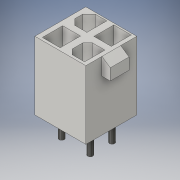
# Autodesk Inventor part: Molex_MiniFitJR_4Pos
Saved by Autodesk Inventor 2016 (Build 200138000, 138)
## iProperties
Created: 2016-09-29
Part Number: Molex_MiniFitJR_4Pos
Material: Generic
Document SubType Name: Modeling
Designer: jfixelle
Density: 1 g/cm^3
Appearance: White
Author: jfixelle
Autodesk Inventor part; units mm, degrees
ref_plane "YZ Plane" through (0, 0, 0) normal (1, 0, 0) x (0, 1, 0)
ref_plane "XZ Plane" through (0, 0, 0) normal (0, 1, 0) x (-1, 0, 0)
ref_plane "XY Plane" through (0, 0, 0) normal (0, 0, 1) x (1, 0, 0)
sketch "Sketch1" plane through (0, 0, 0) normal (0, 1, 0) x (-1, 0, 0)
  line L0 (4.9, 4.9) -> (-4.9, 4.9)
  line L1 (-4.9, 4.9) -> (-4.9, -4.9)
  line L2 (-4.9, -4.9) -> (4.9, -4.9)
  line L3 (4.9, -4.9) -> (4.9, 4.9)
  point P0 (0, 0)
  dimension "d0" = 9.8
  dimension "d1" = 9.8
  dimension "d2" = 4.9
  dimension "d3" = 4.9
  constraints: 8 end point, 2 parallel, 1 horizontal, 1 perpendicular
  measures "d0" distance of L2.end L0.start
  measures "d1" distance of L1.end L2.end
  measures "d2" distance from line of point (0, 0) L2
  measures "d3" distance from line of point (0, 0) L3
extrude "Extrusion1" add sketch "Sketch1" along normal blind 13.1
sketch "Sketch2" plane through (0, 0, 0) normal (0, 0, 1) x (1, 0, 0)
  line L0 (-4.9, 13.1) -> (4.9, 13.1) projected
  line L1 (4.9, 13.1) -> (6.5, 12.0007)
  line L2 (6.5, 12.0007) -> (6.5, 9.8)
  line L3 (6.5, 9.8) -> (4.9, 9.8)
  line L4 (4.9, 9.8) -> (4.9, 13.1)
  line L5 (4.9, 0) -> (4.9, 13.1) projected
  point P0 (0, 0)
  dimension "d6" = 3.3
  dimension "d7" = 1.6
  constraints: 8 end point, 2 perpendicular, 2 point on line
  measures "d6" distance from line of L3 L4.end
  measures "d7" distance of L2.end L3.end
extrude "Extrusion2" add sketch "Sketch2" along normal mid plane 3.6
sketch "Sketch3" plane through (0, 13.1, 0) normal (0, 1, 0) x (1, 0, 0)
  line L0 (-3.9809, -4.385) -> (-0.5456, -4.385)
  line L1 (-0.5456, -4.385) -> (-0.5456, -0.4741)
  line L2 (-0.5456, -0.4741) -> (-3.9809, -0.4741)
  line L3 (-3.9809, -0.4741) -> (-3.9809, -4.385)
  line L4 (0.8079, 0.7571) -> (4.1425, 0.7571)
  line L5 (4.1425, 0.7571) -> (4.1425, 4.5726)
  line L6 (4.1425, 4.5726) -> (0.8079, 4.5726)
  line L7 (0.8079, 4.5726) -> (0.8079, 0.7571)
  line L8 (-0.5456, 0.7571) -> (-3.9809, 0.7571)
  line L9 (-3.9809, 0.7571) -> (-3.9809, 4.5726)
  line L10 (-3.9809, 4.5726) -> (-0.5456, 4.5726)
  line L11 (-0.5456, 4.5726) -> (-0.5456, 0.7571)
  line L12 (0.8079, -4.385) -> (4.1425, -4.385)
  line L13 (4.1425, -4.385) -> (4.1425, -0.4741)
  line L14 (4.1425, -0.4741) -> (0.8079, -0.4741)
  line L15 (0.8079, -0.4741) -> (0.8079, -4.385)
  line L16 (-3.9809, 3.3862) -> (-2.7944, 4.5726)
  line L17 (-3.9809, 1.8506) -> (-2.8874, 0.7571)
  line L18 (0.8079, -3.4193) -> (1.7736, -4.385)
  line L19 (0.8079, -1.3667) -> (1.7005, -0.4741)
  point P0 (0, 0)
  dimension "d10" = 45
  dimension "d11" = 45
  constraints: 40 end point, 16 point on line, 8 parallel, 6 perpendicular, 4 horizontal
  measures "d10" angle of L14 L19
  measures "d11" angle of L12 L18
extrude "Extrusion3" cut sketch "Sketch3" against normal blind 10 contours L3 L2 L1 L0 | L7 L6 L5 L4 | L8 L17 L9 L16 L10 L11 | L18 L15 L19 L14 L13 L12
sketch "Sketch4" plane through (0, 0, 0) normal (0, -1, 0) x (1, 0, 0)
  circle A0 centre (3.05, 2.2) radius 0.5
  line L0 (4.9, 4.9) -> (4.9, -4.9) projected
  line L1 (-4.9, 4.9) -> (4.9, 4.9) projected
  point P0 (0, 0)
  dimension "d15" = 1
  dimension "d16" = 1.85
  dimension "d17" = 2.7
  constraints: 1 centre point
  measures "d15" diameter of A0
  measures "d16" distance from line of L0 A0.centre
  measures "d17" distance from line of L1 A0.centre
extrude "Extrusion4" add sketch "Sketch4" along normal blind 4 and the other way blind 9
pattern_linear "Rectangular Pattern1" count 2 spacing 4.2 along (0, 0, -1) count 2 spacing 5.5 along (-1, 0, 0) of "Extrusion4"
body "Solid1"
